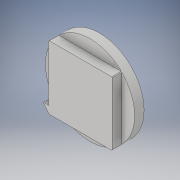
# Autodesk Inventor part: aruco_chip
Saved by Autodesk Inventor 2019 (Build 230136000, 136)
## iProperties
Created: 2024-08-29
Part Number: aruco_chip
Material: Generisch
Document SubType Name: Modeling
Designer: nic
Density: 1 g/cm^3
Appearance: Vorgabe
Author: nic
Autodesk Inventor part; units mm, degrees
ref_plane "YZ Plane" through (0, 0, 0) normal (1, 0, 0) x (0, 1, 0)
ref_plane "XZ Plane" through (0, 0, 0) normal (0, 1, 0) x (-1, 0, 0)
ref_plane "XY Plane" through (0, 0, 0) normal (0, 0, 1) x (1, 0, 0)
sketch "Skizze1" plane through (0, 0, 0) normal (0, 0, 1) x (1, 0, 0)
  circle A0 centre (0, 0) radius 7
  line L0 (-5, 5) -> (5, 5) construction
  line L1 (5, 5) -> (5, -5) construction
  line L2 (5, -5) -> (-5, -5) construction
  line L3 (-5, -5) -> (-5, 5) construction
  line L4 (-5, 5) -> (5, -5) construction
  line L5 (5, 5) -> (-5, -5) construction
  dimension "d0" = 14
  dimension "d1" = 10
  dimension "d2" = 10
  constraints: 12 end point, 2 midpoint, 2 parallel, 1 centre point, 1 coincident, 1 horizontal, 1 perpendicular
  measures "d0" diameter of A0
  measures "d1" distance of L1.end L2.end
  measures "d2" distance of L0.end L1.end
extrude "Extrusion1" add sketch "Skizze1" along normal blind 1.5
sketch "Skizze4" plane through (0, 0, 1.5) normal (0, 0, 1) x (1, 0, 0)
  circle A0 centre (0, 0) radius 7 construction
  line L0 (-5, -5) -> (5, -5)
  line L1 (5, -5) -> (5, 5)
  line L2 (5, 5) -> (-5, 5)
  line L3 (-5, 5) -> (-5, -5)
  line L4 (-5, -5) -> (5, 5) construction
  line L5 (5, -5) -> (-5, 5) construction
  dimension "d9" = 10
  dimension "d10" = 10
  constraints: 12 end point, 2 midpoint, 2 parallel, 1 horizontal, 1 perpendicular
  measures "d9" distance of L2.end L1.end
  measures "d10" distance of L1.end L0.end
extrude "Extrusion3" add sketch "Skizze4" along normal blind 1.5
sketch "Skizze5" plane through (0, 0, 3) normal (0, 0, 1) x (1, 0, 0)
  circle A0 centre (0, 0) radius 7
  circle A1 centre (0, 0) radius 7.3678
  constraints: 2 centre point, 2 coincident
extrude "Extrusion4" cut sketch "Skizze5" against normal through all
sketch "Skizze6" plane through (0, 0, 1.5) normal (0, 0, 1) x (1, 0, 0)
  arc A0 (-5.7802, -3.9484) -> (-5, -4.899) centre (0, 0) ccw
  line L0 (-5, 4.899) -> (-5, -4.899) projected
  line L1 (-5, -3.8099) -> (-5.7802, -3.8099)
  line L2 (-5.7802, -3.8099) -> (-5.7802, -3.9484)
  line L3 (-5.0692, -4.8273) -> (-5, -4.8273)
  line L4 (-5, -4.8273) -> (-5, -3.8099)
  constraints: 9 end point, 3 point on circle, 2 parallel, 2 point on line, 1 centre point, 1 coincident, 1 horizontal, 1 perpendicular
extrude "Extrusion5" add sketch "Skizze6" along normal up to surface (1.5 mm away) contours L2 L1 L0 L3 A0
sketch "Skizze7" plane through (0, 0, 3) normal (0, 0, 1) x (1, 0, 0)
  arc A0 (-5.0692, -4.8273) -> (-5, -4.899) centre (0, 0) ccw projected
  line L0 (-5, -4.8273) -> (-5, -4.899) projected
  line L1 (-5, -4.8273) -> (-5.0692, -4.8273) projected
extrude "Extrusion6" add sketch "Skizze7" against normal up to surface (1.5 mm away)
